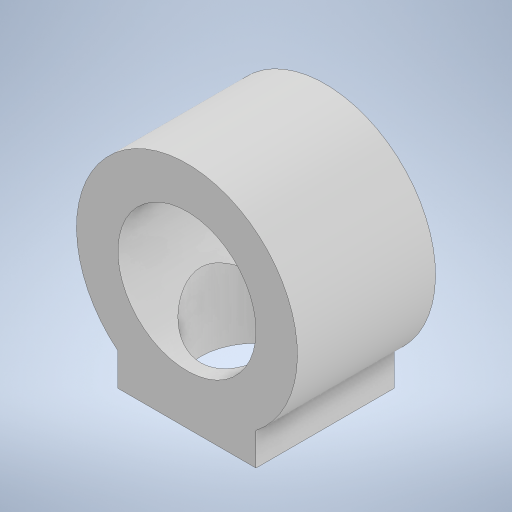
# Autodesk Inventor part: part5
Saved by Autodesk Inventor 2024 (Build 280153000, 153)
## iProperties
Created: 2023-08-22
Part Number: part5
Material: Generic
Document SubType Name: Modeling
Designer: admins
Density: 1 g/cm^3
Appearance: Default
Author: admins
Autodesk Inventor part; units mm, degrees
ref_plane "YZ Plane" through (0, 0, 0) normal (1, 0, 0) x (0, 1, 0)
ref_plane "XZ Plane" through (0, 0, 0) normal (0, 1, 0) x (-1, 0, 0)
ref_plane "XY Plane" through (0, 0, 0) normal (0, 0, 1) x (1, 0, 0)
sketch "Sketch1" plane through (0, 0, 0) normal (0, 1, 0) x (-1, 0, 0)
  line L0 (12.9507, 24.0308) -> (-67.0493, 24.0308)
  line L1 (-67.0493, 24.0308) -> (-67.0493, -25.9692)
  line L2 (-67.0493, -25.9692) -> (12.9507, -25.9692)
  line L3 (12.9507, -25.9692) -> (12.9507, 24.0308)
  point P0 (0, 0)
  dimension "d0" = 80
  dimension "d1" = 50
  constraints: 8 end point, 2 parallel, 1 horizontal, 1 perpendicular
  measures "d0" distance of L2.end L1.end
  measures "d1" distance of L1.end L0.end
extrude "Extrusion1" add sketch "Sketch1" along normal blind 86
sketch "Sketch2" plane through (0, 0, 0) normal (0, -1, 0) x (1, 0, 0)
  circle A0 centre (27.0493, -0.9692) radius 20
  point P0 (0, 0)
  point P1 (67.0493, -25.9692)
  point P2 (-12.9507, 24.0308)
  dimension "d7" = 40
  constraints: 1 centre point
  measures "d7" diameter of A0
sketch "Sketch3" plane through (67.0493, 0, -25.9692) normal (0, 0, -1) x (-1, 0, 0)
  circle A0 centre (40, 43) radius 40
  circle A1 centre (40, 43) radius 25
  line L0 (0, 0) -> (15, 0)
  line L1 (0, 0) -> (80, 0) projected
  line L2 (80, 0) -> (65, 0)
  line L3 (65, 0) -> (65, 11.775)
  line L4 (15, 0) -> (15, 11.775)
  line L5 (0, 86) -> (80, 86) projected
  line L6 (0, 86) -> (80, 86)
  line L7 (80, 86) -> (80, 0)
  line L8 (80, 0) -> (0, 0)
  line L9 (0, 0) -> (0, 86)
  point P0 (67.0493, 0)
  point P1 (0, 43)
  point P2 (80, 43)
  dimension "d10" = 50
  dimension "d15" = 15
  dimension "d16" = 15
  constraints: 16 end point, 3 parallel, 2 centre point, 2 perpendicular, 2 point on circle, 2 point on line, 1 coincident, 1 horizontal
  measures "d10" diameter of A1
  measures "d15" distance of L0.start L0.end
  measures "d16" distance of L1.end L2.end
extrude "Extrusion2" cut sketch "Sketch3" against normal blind 100 contours A1
extrude "Extrusion3" cut sketch "Sketch2" against normal blind 47.6125
extrude "Extrusion4" cut sketch "Sketch3" against normal blind 100 contours L4 L0 L9 A0
extrude "Extrusion5" cut sketch "Sketch3" against normal blind 100 contours A0 L7 L1 L3
extrude "Extrusion6" cut sketch "Sketch3" against normal blind 100 contours L9 L5 L7 A0
body "Solid1"
